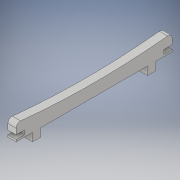
# Autodesk Inventor part: MonsterHolderSupport2
Saved by Autodesk Inventor 2019 (Build 230136000, 136)
## iProperties
Created: 2018-12-04
Part Number: MonsterHolderSupport2
Material: Generic
Document SubType Name: Modeling
Designer: Administrator
Density: 1 g/cm^3
Appearance: Default
Author: Administrator
Autodesk Inventor part; units mm, degrees
ref_plane "YZ Plane" through (0, 0, 0) normal (1, 0, 0) x (0, 1, 0)
ref_plane "XZ Plane" through (0, 0, 0) normal (0, 1, 0) x (-1, 0, 0)
ref_plane "XY Plane" through (0, 0, 0) normal (0, 0, 1) x (1, 0, 0)
sketch "Sketch1" plane through (0, 0, 0) normal (0, 1, 0) x (-1, 0, 0)
  line L0 (0, 0) -> (6.35, 0)
  line L1 (6.35, 0) -> (6.35, -120.65)
  line L2 (6.35, -120.65) -> (0, -120.65)
  line L3 (0, -120.65) -> (0, 0)
  dimension "d0" = 120.65
  dimension "d1" = 6.35
  constraints: 8 end point, 2 parallel, 1 horizontal, 1 perpendicular
  measures "d0" distance of L0.end L1.end
  measures "d1" distance between parallel lines of L3 L1
extrude "Extrusion1" add sketch "Sketch1" along normal blind 12.7
sketch "Sketch2" plane through (0, 0, 0) normal (0, -1, 0) x (1, 0, 0)
  line L0 (0, 0) -> (0, -120.65) projected
  line L1 (-6.35, -120.65) -> (-6.35, 0) projected
  line L2 (0, -12.7) -> (-6.35, -12.7)
  line L3 (-6.35, -12.7) -> (-6.35, -19.05)
  line L4 (-6.35, -19.05) -> (0, -19.05)
  line L5 (0, -19.05) -> (0, -12.7)
  line L6 (0, -101.6) -> (-6.35, -101.6)
  line L7 (-6.35, -101.6) -> (-6.35, -107.95)
  line L8 (-6.35, -107.95) -> (0, -107.95)
  line L9 (0, -107.95) -> (0, -101.6)
  line L10 (-6.35, -120.65) -> (0, -120.65) projected
  line L11 (0, 0) -> (-6.35, 0) projected
  dimension "d4" = 6.35
  dimension "d5" = 12.7
  dimension "d6" = 12.7
  dimension "d7" = 6.35
  constraints: 16 end point, 4 parallel, 4 point on line, 2 horizontal, 2 perpendicular
  measures "d4" distance between parallel lines of L6 L8
  measures "d5" distance between parallel lines of L10 L8
  measures "d6" distance between parallel lines of L11 L2
  measures "d7" distance between parallel lines of L4 L2
extrude "Extrusion2" add sketch "Sketch2" along normal blind 6.35 contours L0 L4 L1 L2 | L0 L8 L1 L6
sketch "Sketch3" plane through (0, 0, -120.65) normal (1, 0, 0) x (0, 0, -1)
  line L0 (-120.65, 0) -> (-120.65, 12.7) projected
  line L1 (-120.65, 4.7625) -> (-114.3, 4.7625)
  line L2 (-114.3, 4.7625) -> (-114.3, 1.5875)
  line L3 (-114.3, 1.5875) -> (-120.65, 1.5875)
  line L4 (-120.65, 1.5875) -> (-120.65, 4.7625)
  line L5 (0, 0) -> (0, 12.7) projected
  line L6 (0, 4.7625) -> (-6.35, 4.7625)
  line L7 (-6.35, 4.7625) -> (-6.35, 1.5875)
  line L8 (-6.35, 1.5875) -> (0, 1.5875)
  line L9 (0, 1.5875) -> (0, 4.7625)
  line L10 (-107.95, 0) -> (-120.65, 0) projected
  dimension "d10" = 6.35
  dimension "d11" = 3.175
  dimension "d12" = 1.5875
  dimension "d13" = 6.35
  constraints: 16 end point, 4 parallel, 4 point on line, 2 horizontal, 2 perpendicular
  measures "d10" distance between parallel lines of L0 L2
  measures "d11" distance between parallel lines of L1 L3
  measures "d12" distance between parallel lines of L10 L3
  measures "d13" distance between parallel lines of L5 L7
extrude "Extrusion3" cut sketch "Sketch3" against normal blind 6.35
sketch "Sketch4" plane through (0, 12.7, 0) normal (1, 0, 0) x (0, 0, -1)
  line L0 (0, -7.9375) -> (0, 0) projected
  line L1 (120.65, -7.9375) -> (120.65, 0) projected
  arc A0 (0, 0) -> (120.65, 0) centre (60.325, 555.5343) ccw
  line L2 (120.65, 0) -> (0, 0) projected
  line L3 (0, 0) -> (120.65, 0)
  point P0 (0, -12.7)
  dimension "d16" = 558.8
  constraints: 2 end point, 2 point on circle, 1 centre point, 1 collinear
  measures "d16" radius of A0
extrude "Extrusion4" cut sketch "Sketch4" against normal blind 6.35
fillet "Fillet1" radius 3.175 2 edges at (-3.175, 12.7, 0) (-3.175, 12.7, -120.65)
body "Solid1"
